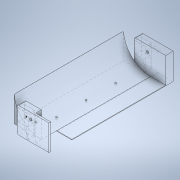
# Autodesk Inventor part: 零件1
Saved by Autodesk Inventor 2020 (Build 240168000, 168)
## iProperties
Created: 2020-12-03
Part Number: 零件1
Material: 常规
Document SubType Name: Sheet Metal
Designer: huang
Density: 1 g/cm^3
Sheet Metal Rule: 默认_mm
Appearance: 默认
Author: huang
## iProperties of the stored document _3D 打印.ipt
Created: 2020-12-07
Part Number: _3D 打印
Material: 常规
Document SubType Name: Modeling
Designer: huang
Density: 1 g/cm^3
Appearance: 默认
Author: huang
Autodesk Inventor part; units mm, degrees
ref_plane "YZ Plane" through (0, 0, 0) normal (1, 0, 0) x (0, 1, 0)
ref_plane "XZ Plane" through (0, 0, 0) normal (0, 1, 0) x (-1, 0, 0)
ref_plane "XY Plane" through (0, 0, 0) normal (0, 0, 1) x (1, 0, 0)
sketch "草图1" plane through (0, 0, 0) normal (0, 1, 0) x (-1, 0, 0)
  line L0 (44.8045, 656.8377) -> (-45.1955, 656.8377)
  line L1 (-45.1955, 656.8377) -> (-45.1955, -101.1623)
  line L2 (-45.1955, -101.1623) -> (44.8045, -101.1623)
  line L3 (44.8045, -101.1623) -> (44.8045, 656.8377)
  point P0 (0, 0)
  dimension "d0" = 90
  dimension "d1" = 758
  constraints: 8 end point, 2 parallel, 1 horizontal, 1 perpendicular
  measures "d0" distance of L1.end L2.end
  measures "d1" distance of L2.end L0.start
extrude "拉伸1" add sketch "草图1" along normal blind 90
sketch "草图3" plane through (-44.8045, 0, 656.8377) normal (0, 0, 1) x (1, 0, 0)
  line L0 (90, 0) -> (90, 90) projected
  circle A0 centre (90, 90) radius 90
  line L1 (0, 0) -> (0, 90) projected
  point P0 (44.8045, 0)
  constraints: 1 horizontal alignment, 1 vertical, 1 other
extrude "拉伸3" cut sketch "草图3" against normal through all
sketch "草图6" plane through (-44.8045, 0, 656.8377) normal (0, 0, 1) x (1, 0, 0)
  arc A0 (0, 90) -> (90, 0) centre (90, 90) ccw projected
  arc A1 (0, 90) -> (90, 0) centre (90, 90) ccw
  line L0 (0, 0) -> (0, 90) projected
  line L1 (0, 90) -> (0, 0)
  line L2 (90, 0) -> (0, 0) projected
  line L3 (0, 0) -> (90, 0)
  constraints: 4 end point, 2 point on circle, 1 centre point, 1 collinear, 1 perpendicular, 1 tangent
extrude "拉伸6" cut sketch "草图6" against normal blind 386
sketch "草图9" plane through (0, 0, 0) normal (0, -1, 0) x (1, 0, 0)
  line L0 (45.1955, -101.1623) -> (-44.8045, -101.1623) projected
  line L1 (-44.8045, -101.1623) -> (45.1955, -101.1623)
  line L2 (45.1955, -101.1623) -> (45.1955, -96.1623)
  line L3 (45.1955, -96.1623) -> (-44.8045, -96.1623)
  line L4 (-44.8045, -96.1623) -> (-44.8045, -101.1623)
  point P0 (0, 0)
  point P1 (43.3955, -101.1623)
  point P2 (-44.8045, 270.8377)
  dimension "d47" = 90
  dimension "d48" = 5
  constraints: 8 end point, 2 parallel, 1 horizontal, 1 perpendicular
  measures "d47" distance of L2.end L3.end
  measures "d48" distance of L1.end L2.end
extrude "拉伸9" add sketch "草图9" against normal blind 85
sketch "草图12" plane through (0, 0, 0) normal (0, -1, 0) x (1, 0, 0)
  line L0 (45.1955, 270.8377) -> (-44.8045, 270.8377) projected
  line L1 (45.1955, 270.8377) -> (45.1955, -96.1623) projected
  line L2 (-44.8045, 270.8377) -> (45.1955, 270.8377)
  line L3 (45.1955, 270.8377) -> (45.1955, 265.8377)
  line L4 (45.1955, 265.8377) -> (-44.8045, 265.8377)
  line L5 (-44.8045, 265.8377) -> (-44.8045, 270.8377)
  point P0 (0, 0)
  point P1 (45.1955, -101.1623)
  dimension "d55" = 5
  constraints: 8 end point, 2 parallel, 1 horizontal, 1 perpendicular, 1 point on line
  measures "d55" distance between parallel lines of L0 L4
extrude "拉伸12" add sketch "草图12" against normal blind 85
sketch "草图14" plane through (45.1955, 0, -101.1623) normal (0, 0, -1) x (-1, 0, 0)
  line L0 (0, 85) -> (0, 65)
  line L1 (0, 65) -> (10, 65)
  circle A0 centre (10, 65) radius 4
  point P0 (45.1955, 0)
  dimension "d49" = 20
  dimension "d51" = 10
  dimension "d52" = 8
  constraints: 4 end point, 1 centre point, 1 coincident, 1 horizontal
  measures "d49" distance of L0.start L0.end
  measures "d51" distance of L0.end L1.end
  measures "d52" diameter of A0
extrude "拉伸14" cut sketch "草图14" along normal mid plane 3000
sketch "草图17" plane through (0, 0, 0) normal (0, -1, 0) x (1, 0, 0)
  line L0 (-44.8045, -101.1623) -> (-44.8045, -121.1623)
  line L1 (-44.8045, -121.1623) -> (55.1955, -121.1623)
  line L2 (-44.6655, 270.8377) -> (45.1955, 270.8377) projected
  line L3 (45.1955, 270.8377) -> (-44.8045, 270.8377)
  line L4 (-44.8045, 270.8377) -> (-44.8045, 290.8377)
  line L5 (-44.8045, 290.8377) -> (45.1955, 290.8377)
  line L6 (-44.8045, -101.1623) -> (55.1955, -101.1623)
  line L7 (55.1955, -101.1623) -> (55.1955, -121.1623)
  line L8 (45.1955, 290.8377) -> (55.1955, 290.8377)
  line L9 (55.1955, 290.8377) -> (55.1955, 270.8377)
  line L10 (45.1955, 270.8377) -> (45.1955, 265.8377) projected
  line L11 (55.1955, 270.8377) -> (45.1955, 270.8377)
  point P0 (0, 0)
  dimension "d64" = 20
  dimension "d65" = 100
  dimension "d66" = 90
  dimension "d67" = 20
  dimension "d105" = 10
  constraints: 20 end point, 4 perpendicular, 3 horizontal, 1 parallel
  measures "d64" distance of L0.start L0.end
  measures "d65" distance of L0.end L1.end
  measures "d66" distance of L4.end L5.end
  measures "d67" distance of L3.end L4.end
  measures "d105" distance of L5.end L8.end
extrude "拉伸17" add sketch "草图17" against normal blind 85
sketch "草图19" plane through (-44.8045, 90, -101.1623) normal (-1, 0, 0) x (0, 0, 1)
  line L0 (392, -90) -> (392, -5) projected
  line L1 (390, -35) -> (390, -55)
  line L2 (390, -54) -> (390, -16)
  line L3 (389, -15) -> (370, -15)
  line L4 (369, -16) -> (369, -54)
  line L5 (370, -55) -> (389, -55)
  line L6 (0, 0) -> (372, 0) projected
  line L7 (186, 0) -> (186, -114.3643)
  line L8 (-20, -90) -> (-20, -5)
  line L9 (-20, -52.5) -> (-18, -35)
  line L10 (-18, -35) -> (-18, -54)
  line L11 (-18, -55) -> (-18, -16)
  line L12 (-17, -15) -> (2, -15)
  line L13 (3, -16) -> (3, -54)
  line L14 (2, -55) -> (-17, -55)
  arc A0 (369, -54) -> (370, -55) centre (370, -54) ccw
  arc A1 (389, -55) -> (390, -54) centre (389, -54) ccw
  arc A2 (390, -16) -> (389, -15) centre (389, -16) ccw
  arc A3 (370, -15) -> (369, -16) centre (370, -16) ccw
  arc A4 (2, -55) -> (3, -54) centre (2, -54) ccw
  arc A5 (-18, -54) -> (-17, -55) centre (-17, -54) ccw
  arc A6 (3, -16) -> (2, -15) centre (2, -16) ccw
  arc A7 (-17, -15) -> (-18, -16) centre (-17, -16) ccw
  line L15 (372, -5) -> (392, -5) projected
  point P0 (101.1623, -90)
  point P1 (390, -15)
  point P2 (369, -15)
  point P3 (369, -55)
  point P4 (-18, -15)
  point P5 (3, -15)
  point P6 (3, -55)
  point P7 (390, -54)
  dimension "d76" = 20
  dimension "d77" = 40
  dimension "d79" = 21
  dimension "d82" = 1
  dimension "d90" = 10
  constraints: 26 end point, 18 point on line, 16 point on circle, 16 tangent, 8 centre point, 7 equal radius, 7 symmetric about line, 2 vertical, 1 horizontal, 1 midpoint, 1 parallel, 1 perpendicular
  measures "d76" distance of L1.start L1.end
  measures "d77" distance of L1.end point (390, -15)
  measures "d79" distance of point (390, -15) point (369, -15)
  measures "d82" radius of A0
  measures "d90" distance between parallel lines of L3 L15
extrude "拉伸19" cut sketch "草图19" against normal blind 70
sketch "草图20" plane through (-44.8045, 90, -101.1623) normal (-1, 0, 0) x (0, 0, 1)
  line L0 (392, -90) -> (392, -5) projected
  line L1 (372, -5) -> (367, -5) projected
  line L2 (392, -90) -> (367, -90)
  line L3 (367, -90) -> (367, -5)
  line L4 (367, -5) -> (392, -5)
  line L5 (392, -5) -> (392, -90)
  line L6 (-20, -90) -> (-20, -5) projected
  line L7 (5, -5) -> (5, -90) projected
  line L8 (-20, -90) -> (5, -90)
  line L9 (5, -90) -> (5, -5)
  line L10 (5, -5) -> (-20, -5)
  line L11 (-20, -5) -> (-20, -90)
  point P0 (101.1623, -90)
  point P1 (-20, -5)
  point P2 (5, -90)
  constraints: 16 end point, 4 parallel, 2 horizontal, 2 perpendicular
extrude "拉伸20" cut sketch "草图20" against normal blind 35
sketch "草图21" plane through (45.1955, 0, 290.8377) normal (0, 0, 1) x (1, 0, 0)
  line L0 (-55, 85) -> (10, 85) projected
  line L1 (-55, 85) -> (-150.5721, 85)
  line L2 (-150.5721, 85) -> (-150.5721, 126.2482)
  line L3 (-150.5721, 126.2482) -> (-55, 126.2482)
  line L4 (-55, 126.2482) -> (-55, 85)
  point P0 (-45.1955, 0)
  point P1 (0, 85)
  constraints: 8 end point, 2 parallel, 1 horizontal, 1 perpendicular
extrude "拉伸21" cut sketch "草图21" against normal through all
sketch "草图24" plane through (45.1955, 0, -96.1623) normal (1, 0, 0) x (0, 0, -1)
  line L0 (5, 0) -> (5, 85) projected
  line L1 (0, 0) -> (0, 85) projected
  line L2 (5, 0) -> (0, 0)
  line L3 (0, 0) -> (0, 85)
  line L4 (0, 85) -> (5, 85)
  line L5 (5, 85) -> (5, 0)
  point P0 (-96.1623, 0)
  constraints: 8 end point, 2 parallel, 1 horizontal, 1 perpendicular
extrude "拉伸24" add sketch "草图24" along normal blind 10
fillet "圆角1" radius 5 2 edges at (-44.735, 85, 265.8377) (-44.735, 85, -96.1623)
fillet "圆角2" radius 5 4 edges at (-9.8045, 85, -108.6623) (-9.8045, 85, 278.3377) (-9.8045, 0, -108.6623) (-9.8045, 0, 278.3377)
sketch "草图30" plane through (45.1955, 0, 265.8377) normal (1, 0, 0) x (0, 0, -1)
  line L0 (-5, 85) -> (0, 85) projected
  line L1 (-5, 0) -> (0, 0)
  line L2 (0, 0) -> (0, 85)
  line L3 (0, 85) -> (-5, 85)
  line L4 (-5, 85) -> (-5, 0)
  point P0 (265.8377, 0)
  constraints: 8 end point, 2 parallel, 1 horizontal, 1 perpendicular
extrude "拉伸29" add sketch "草图30" along normal blind 10
sketch "草图32" plane through (55.1955, 0, -96.1623) normal (1, 0, 0) x (0, 0, -1)
  line L0 (-362, 0) -> (-387, 0) projected
  line L1 (-374.5, 0) -> (-311, 0)
  line L2 (25, 0) -> (0, 0) projected
  line L3 (25, 0) -> (-311, 0)
  line L4 (-311, 0) -> (-311, -2)
  line L5 (-311, -2) -> (25, -2)
  line L6 (25, 5) -> (25, 0) projected
  line L7 (25, -2) -> (25, 0)
  line L8 (25, 0) -> (25, -2)
  line L9 (-387, 0) -> (-381, 0)
  line L10 (-362, 0) -> (-387, 0) projected
  point P0 (-96.1623, 0)
  dimension "d110" = 2
  dimension "d121" = 6
  dimension "d122" = 70
  constraints: 14 end point, 2 horizontal, 1 collinear, 1 midpoint, 1 perpendicular, 1 point on line, 1 vertical
  measures "d110" distance of L1.end L4.end
  measures "d121" distance of L0.end L9.end
  measures "d122" distance of L1.end L9.end
extrude "拉伸30" add sketch "草图32" along normal blind 40 and the other way blind 10
sketch "草图33" plane through (55.1955, 0, 290.8377) normal (1, 0, 0) x (0, 0, -1)
  line L0 (0, 85) -> (25, 85) projected
  line L1 (25, 18.761) -> (25, 0) projected
  line L2 (0, 85) -> (25, 85)
  line L3 (25, 85) -> (25, 0)
  line L4 (25, 0) -> (0, 0)
  line L5 (0, 0) -> (0, 85)
  line L6 (412, 0) -> (412, -2) projected
  line L7 (387, 85) -> (412, 85)
  line L8 (412, 85) -> (412, 0)
  line L9 (412, 0) -> (387, 0)
  line L10 (387, 0) -> (387, 85)
  point P0 (290.8377, 0)
  constraints: 16 end point, 4 parallel, 2 horizontal, 2 perpendicular, 1 point on line
extrude "拉伸31" add sketch "草图33" along normal blind 40
sketch "草图34" plane through (95.1955, 0, 290.8377) normal (1, 0, 0) x (0, 0, -1)
  line L0 (25, 0) -> (0, 0) projected
  line L1 (0, 0) -> (6, 0)
  line L2 (6, -19.1205) -> (76, -19.1205)
  line L3 (76, -19.1205) -> (76, 106.1639)
  line L4 (76, 106.1639) -> (6, 106.1639)
  line L5 (6, 106.1639) -> (6, -19.1205)
  point P0 (290.8377, 0)
  dimension "d123" = 6
  dimension "d124" = 70
  constraints: 10 end point, 2 parallel, 1 horizontal, 1 perpendicular, 1 point on line
  measures "d123" distance of L0.end L1.end
  measures "d124" distance of L2.start L2.end
extrude "拉伸32" cut sketch "草图34" against normal blind 50
sketch "草图35" plane through (0, 0, 0) normal (0, -1, 0) x (1, 0, 0)
  line L0 (-4.8045, 290.8377) -> (95.1955, 290.8377) projected
  line L1 (12.3158, 290.8377) -> (12.3158, 280.8377)
  circle A0 centre (12.3158, 280.8377) radius 2
  line L2 (12.3158, 280.8377) -> (12.3158, 84.8377)
  circle A1 centre (12.3158, 84.8377) radius 2
  line L3 (12.3158, 84.8377) -> (12.3158, -111.1623)
  circle A2 centre (12.3158, -111.1623) radius 2
  line L4 (12.3158, 280.8377) -> (12.3158, 84.8377)
  circle A3 centre (12.3158, 182.8377) radius 2
  circle A4 centre (12.3158, -13.1623) radius 2
  point P0 (0, 0)
  dimension "d133" = 10
  dimension "d134" = 4
  dimension "d135" = 196
  dimension "d136" = 4
  dimension "d137" = 196
  dimension "d138" = 4
  dimension "d145" = 4
  dimension "d146" = 4
  constraints: 8 end point, 5 centre point, 3 coincident, 3 vertical, 2 midpoint, 1 collinear, 1 point on line
  measures "d133" distance of L1.start L1.end
  measures "d134" diameter of A0
  measures "d135" distance of L2.start L2.end
  measures "d136" diameter of A1
  measures "d137" distance of L3.start L3.end
  measures "d138" diameter of A2
  measures "d145" diameter of A3
  measures "d146" diameter of A4
extrude "拉伸33" cut sketch "草图35" against normal blind 10
sketch "草图46" plane through (-9.8045, 18.761, -96.1623) normal (0, 0, 1) x (1, 0, 0)
  circle A0 centre (45, 46.239) radius 4 projected
  circle A1 centre (45, 46.239) radius 4
  point P0 (9.8045, -18.761)
  constraints: 1 centre point, 1 coincident
extrude "拉伸43" cut sketch "草图46" along normal mid plane 1000
sketch "草图51" plane through (-9.8045, 5, -121.1623) normal (0, 0, -1) x (-1, 0, 0)
  circle A0 centre (-45, 60) radius 4 projected
  circle A1 centre (-45, 60) radius 13
  circle A2 centre (-45, 60) radius 4
  line L0 (-45, 60) -> (-60.5, 60)
  circle A3 centre (-60.5, 60) radius 2.5
  line L1 (-45, 60) -> (-29.5, 60)
  circle A4 centre (-29.5, 60) radius 2.5
  point P0 (-9.8045, -5)
  dimension "d171" = 26
  dimension "d172" = 8
  dimension "d173" = 15.5
  dimension "d174" = 5
  dimension "d175" = 15.5
  dimension "d176" = 5
  constraints: 4 centre point, 4 coincident, 4 end point, 2 horizontal
  measures "d171" diameter of A1
  measures "d172" diameter of A2
  measures "d173" distance of L0.start L0.end
  measures "d174" diameter of A3
  measures "d175" distance of L0.start L1.end
  measures "d176" diameter of A4
extrude "拉伸48" cut sketch "草图51" against normal blind 10 contours A3 | A4
sketch "草图52" plane through (-9.8045, 5, 290.8377) normal (0, 0, 1) x (1, 0, 0)
  circle A0 centre (45, 60) radius 4 projected
  circle A1 centre (60.5, 60) radius 2.5 projected
  line L0 (45, 60) -> (60.5, 60)
  circle A2 centre (29.5, 60) radius 2.5 projected
  line L1 (60.5, 60) -> (29.5, 60)
  circle A3 centre (60.5, 60) radius 2.5
  circle A4 centre (29.5, 60) radius 2.5
  point P0 (9.8045, -5)
  constraints: 4 end point, 2 centre point, 2 coincident, 2 concentric, 1 collinear, 1 horizontal
extrude "拉伸49" cut sketch "草图52" against normal blind 10 contours A1 | A2
sketch "草图59" plane through (0, 0, 0) normal (0, -1, 0) x (1, 0, 0)
  line L0 (25.1955, 287.8377) -> (25.1955, 288.8377) projected
  line L1 (25.1955, 288.8377) -> (20.1955, 288.8377)
  line L2 (20.1955, 288.8377) -> (20.1955, 268.8377)
  line L3 (25.1955, 268.8377) -> (25.1955, 288.8377)
  line L4 (-9.8045, 267.8377) -> (25.1955, 267.8377) projected
  line L5 (25.1955, 268.8377) -> (25.1955, 267.8377)
  line L6 (25.1955, 267.8377) -> (20.1955, 267.8377)
  line L7 (20.1955, 268.8377) -> (20.1955, 267.8377)
  point P0 (0, 0)
  dimension "d192" = 5
  constraints: 12 end point, 2 perpendicular, 1 horizontal, 1 parallel, 1 point on line, 1 vertical
  measures "d192" distance between parallel lines of L2 L3
extrude "拉伸55" cut sketch "草图59" against normal blind 50
sketch "草图60" plane through (0, 0, 0) normal (0, -1, 0) x (1, 0, 0)
  line L0 (-9.8045, -119.1623) -> (25.1955, -119.1623) projected
  line L1 (-9.8045, -98.1623) -> (25.1955, -98.1623) projected
  line L2 (25.1955, -119.1623) -> (20.1955, -119.1623)
  line L3 (20.1955, -119.1623) -> (20.1955, -98.1623)
  line L4 (20.1955, -98.1623) -> (25.1955, -98.1623)
  line L5 (25.1955, -98.1623) -> (25.1955, -119.1623)
  point P0 (0, 0)
  dimension "d197" = 5
  constraints: 8 end point, 2 parallel, 1 horizontal, 1 perpendicular, 1 point on line
  measures "d197" distance between parallel lines of L3 L5
extrude "拉伸56" cut sketch "草图60" against normal blind 50
equation "\"折弯半径\" = 厚度"
equation "\"折弯释压宽度\" = 厚度"
equation "\"折弯释压深度\" = 0.5 * 厚度"
equation "\"拐角释压尺寸\" = 4 * 厚度"
equation "\"最小余量\" = 2 * 厚度"
equation "\"过渡半径\" = 折弯半径"
equation "\"Jacobi半径尺寸\" = 折弯半径"
equation "\"间隙大小\" = 厚度"
equation "\"厚度\" = 0.5"
